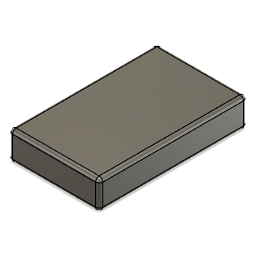
battery (Autodesk Fusion 360 design; units mm, degrees)
Autodesk Fusion 360 part; units mm, degrees
sketch "Sketch1" plane through (0, 0, 0) normal (0, 1, 0) x (1, 0, 0)
  line L0 (0, 0) -> (25, 0)
  line L1 (25, 0) -> (25, 41)
  line L2 (25, 41) -> (0, 41)
  line L3 (0, 41) -> (0, 0)
  dimension "d1" = 25
  dimension "d2" = 41
  constraint horizontal L0
  constraint vertical L1
  constraint horizontal L2
  constraint vertical L3
  constraint coincident L0.start L3.end
  measures "d1" distance of L0.start L0.end
  measures "d2" distance of L0.start L2.end
extrude "Extrude1" add sketch "Sketch1" along normal blind 8
fillet "Fillet1" radius 1 12 edges at (12.5, 8, 0) (25, 8, -20.5) (12.5, 8, -41) (0, 8, -20.5) (25, 0, -20.5) (25, 4, 0) (12.5, 0, 0) (0, 0, -20.5) (0, 4, 0) (0, 4, -41) (12.5, 0, -41) (25, 4, -41)
